Autodesk Inventor part; units mm, degrees
(part 2 of 2)
sketch "Skizze6" plane through (-50, -50, 0) normal (0, 0, -1) x (-1, 0, 0)
  circle A0 centre (-4.394757, 95.405243) radius 1.5
  circle A1 centre (-64.394757, 35.405243) radius 1.5
  circle A2 centre (-4.394757, 35.405243) radius 1.5
  circle A3 centre (-64.394757, 95.405243) radius 1.5
  arc A4 (-9.794757, -7.794757) -> (-7.794757, -9.794757) centre (-7.794757, -7.794757) ccw
  line L0 (10.205243, -9.794757) -> (-7.794757, -9.794757)
  line L1 (10.205243, -10.845267) -> (10.205243, -9.794757)
  arc A5 (9.805243, -11.335165) -> (10.205243, -10.845267) centre (9.705243, -10.845267) ccw
  arc A6 (9.805243, -11.335165) -> (10.205243, -15.294757) centre (10.205243, -13.294757) ccw
  line L2 (20.205243, -15.294757) -> (10.205243, -15.294757)
  arc A7 (20.205243, -15.294757) -> (20.605243, -11.335165) centre (20.205243, -13.294757) ccw
  arc A8 (20.205243, -10.845267) -> (20.605243, -11.335165) centre (20.705243, -10.845267) ccw
  line L3 (20.205243, -9.794757) -> (20.205243, -10.845267)
  line L4 (38.205243, -9.794757) -> (20.205243, -9.794757)
  arc A9 (38.205243, -9.794757) -> (40.205243, -7.794757) centre (38.205243, -7.794757) ccw
  line L5 (40.205243, 10.324875) -> (40.205243, -7.794757)
  line L6 (39.076178, 10.324875) -> (40.205243, 10.324875)
  arc A10 (39.076178, 10.324875) -> (38.677461, 9.984929) centre (39.082965, 9.913117) ccw
  line L7 (38.646985, 9.864261) -> (38.677461, 9.984929)
  arc A11 (34.539143, 10.406652) -> (38.646985, 9.864261) centre (36.602278, 10.205243) ccw
  line L8 (34.539143, 20.205243) -> (34.539143, 10.406652)
  arc A12 (38.67683, 20.623155) -> (34.539143, 20.205243) centre (36.629091, 20.205243) ccw
  arc A13 (38.67683, 20.623155) -> (39.078298, 20.295345) centre (39.078298, 20.705088) ccw
  line L9 (40.205243, 20.295345) -> (39.078298, 20.295345)
  line L10 (40.205243, 38.205243) -> (40.205243, 20.295345)
  arc A14 (40.205243, 38.205243) -> (38.205243, 40.205243) centre (38.205243, 38.205243) ccw
  arc A15 (38.205243, 40.205243) -> (40.205243, 42.205243) centre (38.205243, 42.205243) ccw
  line L11 (40.205243, 60.324875) -> (40.205243, 42.205243)
  line L12 (39.076178, 60.324875) -> (40.205243, 60.324875)
  arc A16 (39.076178, 60.324875) -> (38.677461, 59.984929) centre (39.082965, 59.913117) ccw
  line L13 (38.646985, 59.864261) -> (38.677461, 59.984929)
  arc A17 (34.539143, 60.406652) -> (38.646985, 59.864261) centre (36.602278, 60.205243) ccw
  line L14 (34.539143, 70.205243) -> (34.539143, 60.406652)
  arc A18 (38.67683, 70.623155) -> (34.539143, 70.205243) centre (36.629091, 70.205243) ccw
  arc A19 (38.67683, 70.623155) -> (39.078298, 70.295345) centre (39.078298, 70.705088) ccw
  line L15 (40.205243, 70.295345) -> (39.078298, 70.295345)
  line L16 (40.205243, 88.205243) -> (40.205243, 70.295345)
  arc A20 (40.205243, 88.205243) -> (38.205243, 90.205243) centre (38.205243, 88.205243) ccw
  arc A21 (38.205243, 90.205243) -> (40.205243, 92.205243) centre (38.205243, 92.205243) ccw
  line L17 (40.205243, 110.324875) -> (40.205243, 92.205243)
  line L18 (39.076178, 110.324875) -> (40.205243, 110.324875)
  arc A22 (39.076178, 110.324875) -> (38.677461, 109.984929) centre (39.082965, 109.913117) ccw
  line L19 (38.646985, 109.864261) -> (38.677461, 109.984929)
  arc A23 (34.539143, 110.406652) -> (38.646985, 109.864261) centre (36.602278, 110.205243) ccw
  line L20 (34.539143, 120.205243) -> (34.539143, 110.406652)
  arc A24 (38.67683, 120.623155) -> (34.539143, 120.205243) centre (36.629091, 120.205243) ccw
  arc A25 (38.67683, 120.623155) -> (39.078298, 120.295345) centre (39.078298, 120.705088) ccw
  line L21 (40.205243, 120.295345) -> (39.078298, 120.295345)
  line L22 (40.205243, 138.205243) -> (40.205243, 120.295345)
  arc A26 (40.205243, 138.205243) -> (38.205243, 140.205243) centre (38.205243, 138.205243) ccw
  line L23 (20.085611, 140.205243) -> (38.205243, 140.205243)
  line L24 (20.085611, 139.076178) -> (20.085611, 140.205243)
  arc A27 (20.085611, 139.076178) -> (20.425557, 138.677461) centre (20.497369, 139.082965) ccw
  line L25 (20.546226, 138.646985) -> (20.425557, 138.677461)
  arc A28 (20.003834, 134.539143) -> (20.546226, 138.646985) centre (20.205243, 136.602278) ccw
  line L26 (10.205243, 134.539143) -> (20.003834, 134.539143)
  arc A29 (9.787332, 138.67683) -> (10.205243, 134.539143) centre (10.205243, 136.629091) ccw
  arc A30 (9.787332, 138.67683) -> (10.115141, 139.078298) centre (9.705399, 139.078298) ccw
  line L27 (10.115141, 140.205243) -> (10.115141, 139.078298)
  line L28 (-7.794757, 140.205243) -> (10.115141, 140.205243)
  arc A31 (-7.794757, 140.205243) -> (-9.794757, 138.205243) centre (-7.794757, 138.205243) ccw
  arc A32 (-9.794757, 138.205243) -> (-11.794757, 140.205243) centre (-11.794757, 138.205243) ccw
  line L29 (-29.914389, 140.205243) -> (-11.794757, 140.205243)
  line L30 (-29.914389, 139.076178) -> (-29.914389, 140.205243)
  arc A33 (-29.914389, 139.076178) -> (-29.574443, 138.677461) centre (-29.502631, 139.082965) ccw
  line L31 (-29.453774, 138.646985) -> (-29.574443, 138.677461)
  arc A34 (-29.996166, 134.539143) -> (-29.453774, 138.646985) centre (-29.794757, 136.602278) ccw
  line L32 (-39.794757, 134.539143) -> (-29.996166, 134.539143)
  arc A35 (-40.212668, 138.67683) -> (-39.794757, 134.539143) centre (-39.794757, 136.629091) ccw
  arc A36 (-40.212668, 138.67683) -> (-39.884859, 139.078298) centre (-40.294601, 139.078298) ccw
  line L33 (-39.884859, 140.205243) -> (-39.884859, 139.078298)
  line L34 (-57.794757, 140.205243) -> (-39.884859, 140.205243)
  arc A37 (-57.794757, 140.205243) -> (-59.794757, 138.205243) centre (-57.794757, 138.205243) ccw
  arc A38 (-59.794757, 138.205243) -> (-61.794757, 140.205243) centre (-61.794757, 138.205243) ccw
  line L35 (-79.914389, 140.205243) -> (-61.794757, 140.205243)
  line L36 (-79.914389, 139.076178) -> (-79.914389, 140.205243)
  arc A39 (-79.914389, 139.076178) -> (-79.574443, 138.677461) centre (-79.502631, 139.082965) ccw
  line L37 (-79.453774, 138.646985) -> (-79.574443, 138.677461)
  arc A40 (-79.996166, 134.539143) -> (-79.453774, 138.646985) centre (-79.794757, 136.602278) ccw
  line L38 (-89.794757, 134.539143) -> (-79.996166, 134.539143)
  arc A41 (-90.212668, 138.67683) -> (-89.794757, 134.539143) centre (-89.794757, 136.629091) ccw
  arc A42 (-90.212668, 138.67683) -> (-89.884859, 139.078298) centre (-90.294601, 139.078298) ccw
  line L39 (-89.884859, 140.205243) -> (-89.884859, 139.078298)
  line L40 (-107.794757, 140.205243) -> (-89.884859, 140.205243)
  arc A43 (-107.794757, 140.205243) -> (-109.794757, 138.205243) centre (-107.794757, 138.205243) ccw
  line L41 (-109.794757, 120.205243) -> (-109.794757, 138.205243)
  line L42 (-110.845267, 120.205243) -> (-109.794757, 120.205243)
  arc A44 (-111.335165, 120.605243) -> (-110.845267, 120.205243) centre (-110.845267, 120.705243) ccw
  arc A45 (-111.335165, 120.605243) -> (-115.294757, 120.205243) centre (-113.294757, 120.205243) ccw
  line L43 (-115.294757, 110.205243) -> (-115.294757, 120.205243)
  arc A46 (-115.294757, 110.205243) -> (-111.335165, 109.805243) centre (-113.294757, 110.205243) ccw
  arc A47 (-110.845267, 110.205243) -> (-111.335165, 109.805243) centre (-110.845267, 109.705243) ccw
  line L44 (-109.794757, 110.205243) -> (-110.845267, 110.205243)
  line L45 (-109.794757, 92.205243) -> (-109.794757, 110.205243)
  arc A48 (-109.794757, 92.205243) -> (-107.794757, 90.205243) centre (-107.794757, 92.205243) ccw
  arc A49 (-107.794757, 90.205243) -> (-109.794757, 88.205243) centre (-107.794757, 88.205243) ccw
  line L46 (-109.794757, 70.205243) -> (-109.794757, 88.205243)
  line L47 (-110.845267, 70.205243) -> (-109.794757, 70.205243)
  arc A50 (-111.335165, 70.605243) -> (-110.845267, 70.205243) centre (-110.845267, 70.705243) ccw
  arc A51 (-111.335165, 70.605243) -> (-115.294757, 70.205243) centre (-113.294757, 70.205243) ccw
  line L48 (-115.294757, 60.205243) -> (-115.294757, 70.205243)
  arc A52 (-115.294757, 60.205243) -> (-111.335165, 59.805243) centre (-113.294757, 60.205243) ccw
  arc A53 (-110.845267, 60.205243) -> (-111.335165, 59.805243) centre (-110.845267, 59.705243) ccw
  line L49 (-109.794757, 60.205243) -> (-110.845267, 60.205243)
  line L50 (-109.794757, 42.205243) -> (-109.794757, 60.205243)
  arc A54 (-109.794757, 42.205243) -> (-107.794757, 40.205243) centre (-107.794757, 42.205243) ccw
  arc A55 (-107.794757, 40.205243) -> (-109.794757, 38.205243) centre (-107.794757, 38.205243) ccw
  line L51 (-109.794757, 20.205243) -> (-109.794757, 38.205243)
  line L52 (-110.845267, 20.205243) -> (-109.794757, 20.205243)
  arc A56 (-111.335165, 20.605243) -> (-110.845267, 20.205243) centre (-110.845267, 20.705243) ccw
  arc A57 (-111.335165, 20.605243) -> (-115.294757, 20.205243) centre (-113.294757, 20.205243) ccw
  line L53 (-115.294757, 10.205243) -> (-115.294757, 20.205243)
  arc A58 (-115.294757, 10.205243) -> (-111.335165, 9.805243) centre (-113.294757, 10.205243) ccw
  arc A59 (-110.845267, 10.205243) -> (-111.335165, 9.805243) centre (-110.845267, 9.705243) ccw
  line L54 (-109.794757, 10.205243) -> (-110.845267, 10.205243)
  line L55 (-109.794757, -7.794757) -> (-109.794757, 10.205243)
  arc A60 (-109.794757, -7.794757) -> (-107.794757, -9.794757) centre (-107.794757, -7.794757) ccw
  line L56 (-89.794757, -9.794757) -> (-107.794757, -9.794757)
  line L57 (-89.794757, -10.845267) -> (-89.794757, -9.794757)
  arc A61 (-90.194757, -11.335165) -> (-89.794757, -10.845267) centre (-90.294757, -10.845267) ccw
  arc A62 (-90.194757, -11.335165) -> (-89.794757, -15.294757) centre (-89.794757, -13.294757) ccw
  line L58 (-79.794757, -15.294757) -> (-89.794757, -15.294757)
  arc A63 (-79.794757, -15.294757) -> (-79.394757, -11.335165) centre (-79.794757, -13.294757) ccw
  arc A64 (-79.794757, -10.845267) -> (-79.394757, -11.335165) centre (-79.294757, -10.845267) ccw
  line L59 (-79.794757, -9.794757) -> (-79.794757, -10.845267)
  line L60 (-61.794757, -9.794757) -> (-79.794757, -9.794757)
  arc A65 (-61.794757, -9.794757) -> (-59.794757, -7.794757) centre (-61.794757, -7.794757) ccw
  arc A66 (-59.794757, -7.794757) -> (-57.794757, -9.794757) centre (-57.794757, -7.794757) ccw
  line L61 (-39.794757, -9.794757) -> (-57.794757, -9.794757)
  line L62 (-39.794757, -10.845267) -> (-39.794757, -9.794757)
  arc A67 (-40.194757, -11.335165) -> (-39.794757, -10.845267) centre (-40.294757, -10.845267) ccw
  arc A68 (-40.194757, -11.335165) -> (-39.794757, -15.294757) centre (-39.794757, -13.294757) ccw
  line L63 (-29.794757, -15.294757) -> (-39.794757, -15.294757)
  arc A69 (-29.794757, -15.294757) -> (-29.394757, -11.335165) centre (-29.794757, -13.294757) ccw
  arc A70 (-29.794757, -10.845267) -> (-29.394757, -11.335165) centre (-29.294757, -10.845267) ccw
  line L64 (-29.794757, -9.794757) -> (-29.794757, -10.845267)
  line L65 (-11.794757, -9.794757) -> (-29.794757, -9.794757)
  arc A71 (-11.794757, -9.794757) -> (-9.794757, -7.794757) centre (-11.794757, -7.794757) ccw
  circle A72 centre (-105.594757, 100.705243) radius 2.6
  circle A73 centre (-99.294757, 136.005243) radius 2.6
  circle A74 centre (-63.994757, 129.705243) radius 2.6
  circle A75 centre (-70.294757, 94.405243) radius 2.6
  circle A76 centre (-99.294757, 94.405243) radius 2.6
  circle A77 centre (-104.794757, 95.205243) radius 2.425
  circle A78 centre (-104.794757, 135.205243) radius 2.425
  circle A79 centre (-64.794757, 135.205243) radius 2.425
  circle A80 centre (-84.394757, 94.205243) radius 2.5
  circle A81 centre (-105.794757, 115.405243) radius 2.5
  circle A82 centre (-63.994757, 100.705243) radius 2.6
  circle A83 centre (-70.294757, 136.005243) radius 2.6
  circle A84 centre (-105.594757, 129.705243) radius 2.6
  line L66 (-101.794757, 130.205243) -> (-101.794757, 100.205243)
  arc A85 (-99.794757, 132.205243) -> (-101.794757, 130.205243) centre (-99.794757, 130.205243) ccw
  line L67 (-69.794757, 132.205243) -> (-99.794757, 132.205243)
  arc A86 (-67.794757, 130.205243) -> (-69.794757, 132.205243) centre (-69.794757, 130.205243) ccw
  line L68 (-67.794757, 100.205243) -> (-67.794757, 130.205243)
  arc A87 (-69.794757, 98.205243) -> (-67.794757, 100.205243) centre (-69.794757, 100.205243) ccw
  line L69 (-99.794757, 98.205243) -> (-69.794757, 98.205243)
  arc A88 (-101.794757, 100.205243) -> (-99.794757, 98.205243) centre (-99.794757, 100.205243) ccw
  circle A89 centre (-55.594757, 100.705243) radius 2.6
  circle A90 centre (-49.294757, 136.005243) radius 2.6
  circle A91 centre (-13.994757, 129.705243) radius 2.6
  circle A92 centre (-20.294757, 94.405243) radius 2.6
  circle A93 centre (-49.294757, 94.405243) radius 2.6
  circle A94 centre (-54.794757, 95.205243) radius 2.425
  circle A95 centre (-54.794757, 135.205243) radius 2.425
  circle A96 centre (-14.794757, 95.205243) radius 2.425
  circle A97 centre (-14.794757, 135.205243) radius 2.425
  circle A98 centre (-34.394757, 94.205243) radius 2.5
  circle A99 centre (-55.794757, 115.405243) radius 2.5
  circle A100 centre (-13.994757, 100.705243) radius 2.6
  circle A101 centre (-20.294757, 136.005243) radius 2.6
  circle A102 centre (-55.594757, 129.705243) radius 2.6
  line L70 (-51.794757, 130.205243) -> (-51.794757, 100.205243)
  arc A103 (-49.794757, 132.205243) -> (-51.794757, 130.205243) centre (-49.794757, 130.205243) ccw
  line L71 (-19.794757, 132.205243) -> (-49.794757, 132.205243)
  arc A104 (-17.794757, 130.205243) -> (-19.794757, 132.205243) centre (-19.794757, 130.205243) ccw
  line L72 (-17.794757, 100.205243) -> (-17.794757, 130.205243)
  arc A105 (-19.794757, 98.205243) -> (-17.794757, 100.205243) centre (-19.794757, 100.205243) ccw
  line L73 (-49.794757, 98.205243) -> (-19.794757, 98.205243)
  arc A106 (-51.794757, 100.205243) -> (-49.794757, 98.205243) centre (-49.794757, 100.205243) ccw
  line L74 (-1.794757, 130.205243) -> (-1.794757, 100.205243)
  arc A107 (0.205243, 132.205243) -> (-1.794757, 130.205243) centre (0.205243, 130.205243) ccw
  line L75 (30.205243, 132.205243) -> (0.205243, 132.205243)
  arc A108 (32.205243, 130.205243) -> (30.205243, 132.205243) centre (30.205243, 130.205243) ccw
  line L76 (32.205243, 100.205243) -> (32.205243, 130.205243)
  arc A109 (30.205243, 98.205243) -> (32.205243, 100.205243) centre (30.205243, 100.205243) ccw
  line L77 (0.205243, 98.205243) -> (30.205243, 98.205243)
  arc A110 (-1.794757, 100.205243) -> (0.205243, 98.205243) centre (0.205243, 100.205243) ccw
  circle A111 centre (-5.594757, 129.705243) radius 2.6
  circle A112 centre (29.705243, 136.005243) radius 2.6
  circle A113 centre (36.005243, 100.705243) radius 2.6
  circle A114 centre (-5.794757, 115.405243) radius 2.5
  circle A115 centre (15.605243, 94.205243) radius 2.5
  circle A116 centre (35.205243, 135.205243) radius 2.425
  circle A117 centre (35.205243, 95.205243) radius 2.425
  circle A118 centre (-4.794757, 135.205243) radius 2.425
  circle A119 centre (0.705243, 94.405243) radius 2.6
  circle A120 centre (29.705243, 94.405243) radius 2.6
  circle A121 centre (36.005243, 129.705243) radius 2.6
  circle A122 centre (0.705243, 136.005243) radius 2.6
  circle A123 centre (-5.594757, 100.705243) radius 2.6
  circle A124 centre (-105.594757, 0.705243) radius 2.6
  circle A125 centre (-99.294757, 36.005243) radius 2.6
  circle A126 centre (-63.994757, 29.705243) radius 2.6
  circle A127 centre (-70.294757, -5.594757) radius 2.6
  circle A128 centre (-99.294757, -5.594757) radius 2.6
  circle A129 centre (-104.794757, -4.794757) radius 2.425
  circle A130 centre (-104.794757, 35.205243) radius 2.425
  circle A131 centre (-64.794757, -4.794757) radius 2.425
  circle A132 centre (-84.394757, -5.794757) radius 2.5
  circle A133 centre (-105.794757, 15.405243) radius 2.5
  circle A134 centre (-63.994757, 0.705243) radius 2.6
  circle A135 centre (-70.294757, 36.005243) radius 2.6
  circle A136 centre (-105.594757, 29.705243) radius 2.6
  line L78 (-101.794757, 30.205243) -> (-101.794757, 0.205243)
  arc A137 (-99.794757, 32.205243) -> (-101.794757, 30.205243) centre (-99.794757, 30.205243) ccw
  line L79 (-69.794757, 32.205243) -> (-99.794757, 32.205243)
  arc A138 (-67.794757, 30.205243) -> (-69.794757, 32.205243) centre (-69.794757, 30.205243) ccw
  line L80 (-67.794757, 0.205243) -> (-67.794757, 30.205243)
  arc A139 (-69.794757, -1.794757) -> (-67.794757, 0.205243) centre (-69.794757, 0.205243) ccw
  line L81 (-99.794757, -1.794757) -> (-69.794757, -1.794757)
  arc A140 (-101.794757, 0.205243) -> (-99.794757, -1.794757) centre (-99.794757, 0.205243) ccw
  circle A141 centre (-55.594757, 0.705243) radius 2.6
  circle A142 centre (-49.294757, 36.005243) radius 2.6
  circle A143 centre (-13.994757, 29.705243) radius 2.6
  circle A144 centre (-20.294757, -5.594757) radius 2.6
  circle A145 centre (-49.294757, -5.594757) radius 2.6
  circle A146 centre (-54.794757, -4.794757) radius 2.425
  circle A147 centre (-54.794757, 35.205243) radius 2.425
  circle A148 centre (-14.794757, -4.794757) radius 2.425
  circle A149 centre (-14.794757, 35.205243) radius 2.425
  circle A150 centre (-34.394757, -5.794757) radius 2.5
  circle A151 centre (-55.794757, 15.405243) radius 2.5
  circle A152 centre (-13.994757, 0.705243) radius 2.6
  circle A153 centre (-20.294757, 36.005243) radius 2.6
  circle A154 centre (-55.594757, 29.705243) radius 2.6
  line L82 (-51.794757, 30.205243) -> (-51.794757, 0.205243)
  arc A155 (-49.794757, 32.205243) -> (-51.794757, 30.205243) centre (-49.794757, 30.205243) ccw
  line L83 (-19.794757, 32.205243) -> (-49.794757, 32.205243)
  arc A156 (-17.794757, 30.205243) -> (-19.794757, 32.205243) centre (-19.794757, 30.205243) ccw
  line L84 (-17.794757, 0.205243) -> (-17.794757, 30.205243)
  arc A157 (-19.794757, -1.794757) -> (-17.794757, 0.205243) centre (-19.794757, 0.205243) ccw
  line L85 (-49.794757, -1.794757) -> (-19.794757, -1.794757)
  arc A158 (-51.794757, 0.205243) -> (-49.794757, -1.794757) centre (-49.794757, 0.205243) ccw
  line L86 (-51.794757, 80.205243) -> (-51.794757, 50.205243)
  arc A159 (-49.794757, 82.205243) -> (-51.794757, 80.205243) centre (-49.794757, 80.205243) ccw
  line L87 (-19.794757, 82.205243) -> (-49.794757, 82.205243)
  arc A160 (-17.794757, 80.205243) -> (-19.794757, 82.205243) centre (-19.794757, 80.205243) ccw
  line L88 (-17.794757, 50.205243) -> (-17.794757, 80.205243)
  arc A161 (-19.794757, 48.205243) -> (-17.794757, 50.205243) centre (-19.794757, 50.205243) ccw
  line L89 (-49.794757, 48.205243) -> (-19.794757, 48.205243)
  arc A162 (-51.794757, 50.205243) -> (-49.794757, 48.205243) centre (-49.794757, 50.205243) ccw
  circle A163 centre (-55.594757, 79.705243) radius 2.6
  circle A164 centre (-20.294757, 86.005243) radius 2.6
  circle A165 centre (-13.994757, 50.705243) radius 2.6
  circle A166 centre (-55.794757, 65.405243) radius 2.5
  circle A167 centre (-34.394757, 44.205243) radius 2.5
  circle A168 centre (-14.794757, 85.205243) radius 2.425
  circle A169 centre (-14.794757, 45.205243) radius 2.425
  circle A170 centre (-54.794757, 85.205243) radius 2.425
  circle A171 centre (-54.794757, 45.205243) radius 2.425
  circle A172 centre (-49.294757, 44.405243) radius 2.6
  circle A173 centre (-20.294757, 44.405243) radius 2.6
  circle A174 centre (-13.994757, 79.705243) radius 2.6
  circle A175 centre (-49.294757, 86.005243) radius 2.6
  circle A176 centre (-55.594757, 50.705243) radius 2.6
  circle A177 centre (-5.594757, 50.705243) radius 2.6
  circle A178 centre (0.705243, 86.005243) radius 2.6
  circle A179 centre (36.005243, 79.705243) radius 2.6
  circle A180 centre (29.705243, 44.405243) radius 2.6
  circle A181 centre (0.705243, 44.405243) radius 2.6
  circle A182 centre (-4.794757, 45.205243) radius 2.425
  circle A183 centre (-4.794757, 85.205243) radius 2.425
  circle A184 centre (35.205243, 45.205243) radius 2.425
  circle A185 centre (35.205243, 85.205243) radius 2.425
  circle A186 centre (15.605243, 44.205243) radius 2.5
  circle A187 centre (-5.794757, 65.405243) radius 2.5
  circle A188 centre (36.005243, 50.705243) radius 2.6
  circle A189 centre (29.705243, 86.005243) radius 2.6
  circle A190 centre (-5.594757, 79.705243) radius 2.6
  line L90 (-1.794757, 80.205243) -> (-1.794757, 50.205243)
  arc A191 (0.205243, 82.205243) -> (-1.794757, 80.205243) centre (0.205243, 80.205243) ccw
  line L91 (30.205243, 82.205243) -> (0.205243, 82.205243)
  arc A192 (32.205243, 80.205243) -> (30.205243, 82.205243) centre (30.205243, 80.205243) ccw
  line L92 (32.205243, 50.205243) -> (32.205243, 80.205243)
  arc A193 (30.205243, 48.205243) -> (32.205243, 50.205243) centre (30.205243, 50.205243) ccw
  line L93 (0.205243, 48.205243) -> (30.205243, 48.205243)
  arc A194 (-1.794757, 50.205243) -> (0.205243, 48.205243) centre (0.205243, 50.205243) ccw
  line L94 (-101.794757, 80.205243) -> (-101.794757, 50.205243)
  arc A195 (-99.794757, 82.205243) -> (-101.794757, 80.205243) centre (-99.794757, 80.205243) ccw
  line L95 (-69.794757, 82.205243) -> (-99.794757, 82.205243)
  arc A196 (-67.794757, 80.205243) -> (-69.794757, 82.205243) centre (-69.794757, 80.205243) ccw
  line L96 (-67.794757, 50.205243) -> (-67.794757, 80.205243)
  arc A197 (-69.794757, 48.205243) -> (-67.794757, 50.205243) centre (-69.794757, 50.205243) ccw
  line L97 (-99.794757, 48.205243) -> (-69.794757, 48.205243)
  arc A198 (-101.794757, 50.205243) -> (-99.794757, 48.205243) centre (-99.794757, 50.205243) ccw
  circle A199 centre (-105.594757, 79.705243) radius 2.6
  circle A200 centre (-70.294757, 86.005243) radius 2.6
  circle A201 centre (-63.994757, 50.705243) radius 2.6
  circle A202 centre (-105.794757, 65.405243) radius 2.5
  circle A203 centre (-84.394757, 44.205243) radius 2.5
  circle A204 centre (-64.794757, 85.205243) radius 2.425
  circle A205 centre (-64.794757, 45.205243) radius 2.425
  circle A206 centre (-104.794757, 85.205243) radius 2.425
  circle A207 centre (-104.794757, 45.205243) radius 2.425
  circle A208 centre (-99.294757, 44.405243) radius 2.6
  circle A209 centre (-70.294757, 44.405243) radius 2.6
  circle A210 centre (-63.994757, 79.705243) radius 2.6
  circle A211 centre (-99.294757, 86.005243) radius 2.6
  circle A212 centre (-105.594757, 50.705243) radius 2.6
  circle A213 centre (-5.594757, 0.705243) radius 2.6
  circle A214 centre (0.705243, 36.005243) radius 2.6
  circle A215 centre (36.005243, 29.705243) radius 2.6
  circle A216 centre (29.705243, -5.594757) radius 2.6
  circle A217 centre (0.705243, -5.594757) radius 2.6
  circle A218 centre (-4.794757, -4.794757) radius 2.425
  circle A219 centre (35.205243, -4.794757) radius 2.425
  circle A220 centre (35.205243, 35.205243) radius 2.425
  circle A221 centre (15.605243, -5.794757) radius 2.5
  circle A222 centre (-5.794757, 15.405243) radius 2.5
  circle A223 centre (36.005243, 0.705243) radius 2.6
  circle A224 centre (29.705243, 36.005243) radius 2.6
  circle A225 centre (-5.594757, 29.705243) radius 2.6
  line L98 (-1.794757, 30.205243) -> (-1.794757, 0.205243)
  arc A226 (0.205243, 32.205243) -> (-1.794757, 30.205243) centre (0.205243, 30.205243) ccw
  line L99 (30.205243, 32.205243) -> (0.205243, 32.205243)
  arc A227 (32.205243, 30.205243) -> (30.205243, 32.205243) centre (30.205243, 30.205243) ccw
  line L100 (32.205243, 0.205243) -> (32.205243, 30.205243)
  arc A228 (30.205243, -1.794757) -> (32.205243, 0.205243) centre (30.205243, 0.205243) ccw
  line L101 (0.205243, -1.794757) -> (30.205243, -1.794757)
  arc A229 (-1.794757, 0.205243) -> (0.205243, -1.794757) centre (0.205243, 0.205243) ccw
  circle A230 centre (-34.794757, 65.205243) radius 17
  line L102 (-51.794757, 80.205243) -> (-51.794757, 50.205243)
  line L103 (-17.794757, 50.205243) -> (-17.794757, 80.205243)
  point P0 (-50, 50)
  constraints: 3 tangent, 1 centre point
equation "\"d24\" = d23"
equation "\"d25\" = d23"
equation "\"d26\" = d23"
equation "\"d27\" = d23"
equation "\"d28\" = d23"
equation "\"d29\" = d23"
equation "\"d30\" = d23"
body "Solid2"
